Autodesk Fusion 360 part; units mm, degrees
(part 2 of 2)
  arc A548 (60.8258, -81.7071) -> (60.1702, -83.0409) centre (61.6673, -82.9488) ccw
  arc A549 (59.9867, -83.4594) -> (60.1702, -83.0409) centre (59.6711, -83.0716) ccw
  arc A550 (58.7428, -83.7927) -> (59.9867, -83.4594) centre (47.5, -39.3462) ccw
  arc A551 (58.3747, -83.522) -> (58.7428, -83.7927) centre (58.8222, -83.2991) ccw
  arc A552 (58.3747, -83.522) -> (57.14, -82.6947) centre (57.032, -84.1908) ccw
  arc A553 (56.3249, -82.8679) -> (57.14, -82.6947) centre (56.5824, -82.0754) ccw
  arc A554 (56.3249, -82.8679) -> (55.5334, -84.1259) centre (57.032, -84.1908) ccw
  arc A555 (55.3072, -84.523) -> (55.5334, -84.1259) centre (55.0339, -84.1043) ccw
  arc A556 (54.0353, -84.7245) -> (55.3072, -84.523) centre (47.5, -39.3462) ccw
  arc A557 (53.6975, -84.4167) -> (54.0353, -84.7245) centre (54.1659, -84.2418) ccw
  arc A558 (53.6975, -84.4167) -> (52.556, -83.4649) centre (52.2923, -84.9415) ccw
  arc A559 (51.7273, -83.552) -> (52.556, -83.4649) centre (52.0662, -82.7907) ccw
  arc A560 (51.7273, -83.552) -> (50.8087, -84.7204) centre (52.2923, -84.9415) ccw
  arc A561 (50.5422, -85.0916) -> (50.8087, -84.7204) centre (50.3141, -84.6466) ccw
  line L46 (-17.9167, 5.0594) -> (-17.0833, 5.0594)
  line L47 (-52.9167, 5.0594) -> (-52.0833, 5.0594)
  line L48 (-47.9167, 5.0594) -> (-47.0833, 5.0594)
  line L49 (-42.9167, 5.0594) -> (-42.0833, 5.0594)
  line L50 (-37.9167, 5.0594) -> (-37.0833, 5.0594)
  line L51 (-32.9167, 5.0594) -> (-32.0833, 5.0594)
  line L52 (-27.9167, 5.0594) -> (-27.0833, 5.0594)
  line L53 (-22.9167, 5.0594) -> (-22.0833, 5.0594)
  line L54 (-12.9167, 5.0594) -> (-12.0833, 5.0594)
  line L55 (-7.9167, 5.0594) -> (-7.0833, 5.0594)
  line L56 (-2.9167, 5.0594) -> (-2.0833, 5.0594)
  line L57 (2.0833, 5.0594) -> (2.9167, 5.0594)
  line L58 (7.0833, 5.0594) -> (7.9167, 5.0594)
  line L59 (12.0833, 5.0594) -> (12.9167, 5.0594)
  line L60 (17.0833, 5.0594) -> (17.9167, 5.0594)
  line L61 (22.0833, 5.0594) -> (22.9167, 5.0594)
  dimension "d25" = 5
  dimension "d26" = 0
  constraint coincident A319.end A320.end
  constraint coincident A320.start A321.start
extrude "Extrude2" cut sketch "Sketch2" against normal up to surface (36 mm away) contours L3 A320 L46 | L3 A320 L46 | L2 L3 A320 A321 A322 | L1 L2 A353 A354 A355 | L2 A323 A324 A325 A326 A327 | L2 A348 A349 A350 A351 A352 | L2 A328 A329 A330 A331 A332 | A325 L54 | L2 A343 A344 A345 A346 A347 | A350 L59 | L2 A333 A334 A335 A336 A337 | A330 L55 | L2 A338 A339 A340 A341 A342 | A345 L58 | A335 L56 | A340 L57 | A0 L4 A1 L5
move_face "OffsetFaces1" [suppressed]
sketch "Sketch3" plane through (0, 0, 0) normal (0, 0, -1) x (1, 0, 0)
  circle A0 centre (-12.5, -13) radius 2.25
  circle A1 centre (-12.5, 13) radius 2.25
  circle A2 centre (12.5, -13) radius 2.25
  circle A3 centre (12.5, 13) radius 2.25
  line L0 (17.5, -18) -> (17.5, 18)
  line L1 (17.5, 18) -> (-17.5, 18)
  line L2 (-17.5, 18) -> (-17.5, -18)
  line L3 (-17.5, -18) -> (17.5, -18)
  line L4 (12.7, 12.7) -> (-12.7, 12.7) construction
  line L5 (-12.7, 12.7) -> (-12.7, -12.7) construction
  line L6 (-12.7, -12.7) -> (12.7, -12.7) construction
  line L7 (12.7, -12.7) -> (12.7, 12.7) construction
  line L8 (12.7, 12.7) -> (-12.7, -12.7) construction
  line L9 (-12.7, 12.7) -> (12.7, -12.7) construction
  dimension "d30" = 25.4
  dimension "d31" = 25.4
  constraint horizontal L4
  constraint perpendicular L4 L5
  constraint parallel L4 L6
  constraint parallel L5 L7
  constraint coincident L8 origin
  constraint coincident L9 origin
  measures "d30" distance of L5.end L6.end
  measures "d31" distance of L4.end L5.end
hole "Hole1" at (-12.7, -12.7, 0) at (12.7, -12.7, 0) at (12.7, 12.7, 0) at (-12.7, 12.7, 0) direction (0, 0, 1) diameter 5.613 end through all
equation "Type = 'HTD5-20mm'"
equation "_W = 20 mm"
equation "_A = 35 mm"
equation "_B = 36 mm"
equation "_P = 26 mm"
equation "_L = 25 mm"
equation "_T = 6.5 mm"
equation "_h = 2.1 mm"
equation "_d = 4.5 mm"
equation "d10 = _A"
equation "d11 = _B"
equation "d13 = _L"
equation "d14 = _P"
equation "d15 = _d"
equation "d16 = _T"
equation "d22 = -_h + 0.771 mm"
equation "THIN_AMT = 2.5 mm" comment "Amount to trim down back of plate"
equation "d37 = -THIN_AMT"
